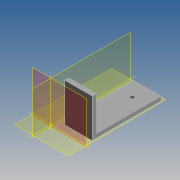
# Autodesk Inventor part: P005_supportCapteursTripod
Saved by Autodesk Inventor 2020 (Build 240168000, 168)
## iProperties
Created: 2021-10-05
Part Number: P005_supportCapteursTripod
Material: Générique
Document SubType Name: Modeling
Designer: gabri
Density: 1 g/cm^3
Appearance: Par défaut
Author: gabri
Autodesk Inventor part; units mm, degrees
sketch "Esquisse2" plane through (0, 0, 0) normal (0, 0, 1) x (1, 0, 0)
  line L0 (10, 110) -> (50, 110)
  line L1 (50, 110) -> (50, 10)
  line L2 (50, 10) -> (10, 10)
  line L3 (10, 10) -> (10, 110)
  line L4 (0, 132) -> (0, -22) construction
  line L5 (-10, 0) -> (60, 0) construction
  point P0 (0, 0)
  dimension "d0" = 40
  dimension "d1" = 100
  dimension "d2" = 10
  dimension "d3" = 10
  constraints: 8 end point, 2 parallel, 1 horizontal, 1 perpendicular
  measures "d0" distance between parallel lines of L1 L3
  measures "d1" distance of L0.end L1.end
  measures "d2" distance between parallel lines of L4 L3
  measures "d3" distance between parallel lines of L5 L2
extrude "Extrusion1" add sketch "Esquisse2" along normal blind 6
sketch "Esquisse3" plane through (0, 0, 6) normal (0, 0, 1) x (1, 0, 0)
  line L0 (50, 10) -> (50, 110) construction
  line L1 (50, 110) -> (10, 110) construction
  line L2 (10, 110) -> (10, 10) construction
  line L3 (10, 10) -> (50, 10) construction
  line L4 (50, 10) -> (10, 10)
  line L5 (10, 10) -> (10, 16)
  line L6 (10, 16) -> (50, 16)
  line L7 (50, 16) -> (50, 10)
  point P0 (0, 0)
  dimension "d6" = 6
  constraints: 8 end point, 2 parallel, 1 horizontal, 1 perpendicular, 1 point on line
  measures "d6" distance between parallel lines of L3 L6
extrude "Extrusion2" add sketch "Esquisse3" along normal blind 50
sketch "Esquisse4" plane through (0, 0, 0) normal (0, 0, -1) x (-1, 0, 0)
  line L0 (-50, 10) -> (-50, 110) construction
  line L1 (-10, 10) -> (-50, 10) construction
  line L2 (-10, 110) -> (-10, 10) construction
  line L3 (-50, 110) -> (-10, 110) construction
  line L4 (-10, 110) -> (-50, 110) construction
  line L5 (-50, 110) -> (-50, 65) construction
  line L6 (-50, 65) -> (-10, 65) construction
  line L7 (-10, 65) -> (-10, 110) construction
  circle A0 centre (-30, 87.5) radius 3
  point P0 (0, 0)
  dimension "d9" = 45
  dimension "d10" = 6
  dimension "d11" = 20
  dimension "d12" = 22.5
  constraints: 8 end point, 2 parallel, 1 centre point, 1 coincident, 1 horizontal, 1 perpendicular, 1 point on line
  measures "d9" distance between parallel lines of L6 L3
  measures "d10" diameter of A0
  measures "d11" distance from line of L2 A0.centre
  measures "d12" distance from line of L3 A0.centre
hole "Perçage1" at (30, 87.5, 0) direction (0, 0, 1) diameter 6 depth 6 tip angle 118
